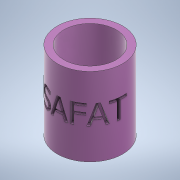
# Autodesk Inventor part: Repujado 2
Saved by Autodesk Inventor 2021 (Build 250183000, 183)
## iProperties
Created: 2021-01-13
Part Number: Repujado 2
Material: Genérico
Document SubType Name: Modeling
Designer: yosaf
Density: 1 g/cm^3
Appearance: Valor por defecto
Author: yosaf
Autodesk Inventor part; units mm, degrees
ref_plane "YZ Plane" through (0, 0, 0) normal (1, 0, 0) x (0, 1, 0)
ref_plane "XZ Plane" through (0, 0, 0) normal (0, 1, 0) x (-1, 0, 0)
sketch "Boceto1" plane through (0, 0, 0) normal (0, 1, 0) x (-1, 0, 0)
  circle A0 centre (0, 0) radius 25
  dimension "d0" = 50
  constraints: 1 centre point, 1 coincident
  measures "d0" diameter of A0
extrude "Extrusión1" add sketch "Boceto1" along normal blind 60
ref_plane "Plano de trabajo1" through (0, 0, 25) normal (0, 0, 1) x (1, 0, 0)
sketch "Boceto2" plane through (0, 0, 25) normal (0, 0, 1) x (1, 0, 0)
  line L0 (-43.1881, 39.0863) -> (43.2155, 39.0863) construction
  line L1 (43.2155, 39.0863) -> (43.2155, 23.3552) construction
  line L2 (43.2155, 23.3552) -> (-43.1881, 23.3552) construction
  line L3 (-43.1881, 23.3552) -> (-43.1881, 39.0863) construction
  line L4 (-31.1662, 38.7702) -> (-36.2351, 30.4072)
  line L5 (-36.2351, 30.4072) -> (-36.2351, 23.7702)
  line L6 (-36.2351, 23.7702) -> (-38.2286, 23.7702)
  line L7 (-38.2286, 23.7702) -> (-38.2286, 30.2005)
  line L8 (-38.2286, 30.2005) -> (-43.2975, 38.7702)
  line L9 (-43.2975, 38.7702) -> (-41.0852, 38.7702)
  line L10 (-41.0852, 38.7702) -> (-37.2197, 32.1697)
  line L11 (-37.2197, 32.1697) -> (-33.2813, 38.7702)
  line L12 (-33.2813, 38.7702) -> (-31.1662, 38.7702)
  spline S0 degree 2 poles (-19.1687, 37.0563) (-18.3178, 36.0595) (-17.3696, 33.1422) (-17.3696, 31.2702) knots 0 0 0 1 2 2 2
  spline S1 degree 2 poles (-17.3696, 31.2702) (-17.3696, 29.4469) (-18.2935, 26.4931) (-19.1687, 25.4963) knots 0 0 0 1 2 2 2
  spline S2 degree 2 poles (-19.1687, 25.4963) (-20.0925, 24.4509) (-22.5358, 23.4542) (-24.0066, 23.4542) knots 0 0 0 1 2 2 2
  spline S3 degree 2 poles (-24.0066, 23.4542) (-25.526, 23.4542) (-27.9572, 24.4874) (-28.8445, 25.4963) knots 0 0 0 1 2 2 2
  spline S4 degree 2 poles (-28.8445, 25.4963) (-29.7076, 26.4931) (-30.6314, 29.4226) (-30.6314, 31.2702) knots 0 0 0 1 2 2 2
  spline S5 degree 2 poles (-30.6314, 31.2702) (-30.6314, 33.1543) (-29.6954, 36.0231) (-28.8324, 37.0563) knots 0 0 0 1 2 2 2
  spline S6 degree 2 poles (-28.8324, 37.0563) (-27.9572, 38.053) (-25.5139, 39.0863) (-24.0066, 39.0863) knots 0 0 0 1 2 2 2
  spline S7 degree 2 poles (-24.0066, 39.0863) (-22.475, 39.0863) (-20.0196, 38.0166) (-19.1687, 37.0563) knots 0 0 0 1 2 2 2
  spline S8 degree 2 poles (-19.4482, 31.2702) (-19.4482, 32.7532) (-20.0925, 35.0506) (-20.676, 35.8043) knots 0 0 0 1 2 2 2
  spline S9 degree 2 poles (-20.676, 35.8043) (-21.2716, 36.5822) (-22.949, 37.3602) (-23.9944, 37.3602) knots 0 0 0 1 2 2 2
  spline S10 degree 2 poles (-23.9944, 37.3602) (-25.0763, 37.3602) (-26.7051, 36.6065) (-27.3251, 35.8043) knots 0 0 0 1 2 2 2
  spline S11 degree 2 poles (-27.3251, 35.8043) (-27.9207, 35.0385) (-28.5528, 32.7289) (-28.5528, 31.2702) knots 0 0 0 1 2 2 2
  spline S12 degree 2 poles (-28.5528, 31.2702) (-28.5528, 28.3164) (-26.073, 25.1803) (-23.9944, 25.1803) knots 0 0 0 1 2 2 2
  spline S13 degree 2 poles (-23.9944, 25.1803) (-21.9158, 25.1803) (-19.4482, 28.3164) (-19.4482, 31.2702) knots 0 0 0 1 2 2 2
  spline S14 degree 2 poles (-11.0001, 23.5028) (-12.629, 23.5028) (-14.9142, 24.1835) (-15.9231, 24.6697) knots 0 0 0 1 2 2 2
  line L13 (-15.9231, 24.6697) -> (-15.9231, 27.1738)
  line L14 (-15.9231, 27.1738) -> (-15.7772, 27.1738)
  spline S15 degree 2 poles (-15.7772, 27.1738) (-14.7926, 26.25) (-12.3008, 25.2289) (-11.146, 25.2289) knots 0 0 0 1 2 2 2
  spline S16 degree 2 poles (-11.146, 25.2289) (-9.4928, 25.2289) (-7.8032, 26.6025) (-7.8032, 27.7329) knots 0 0 0 1 2 2 2
  spline S17 degree 2 poles (-7.8032, 27.7329) (-7.8032, 28.6325) (-8.6905, 29.7508) (-9.6508, 30.0304) knots 0 0 0 1 2 2 2
  spline S18 degree 2 poles (-9.6508, 30.0304) (-10.3437, 30.2248) (-11.4985, 30.4923) (-12.3615, 30.7111) knots 0 0 0 1 2 2 2
  spline S19 degree 2 poles (-12.3615, 30.7111) (-13.1395, 30.9177) (-14.3672, 31.5376) (-14.8413, 32.036) knots 0 0 0 1 2 2 2
  spline S20 degree 2 poles (-14.8413, 32.036) (-15.3032, 32.5344) (-15.8137, 33.8715) (-15.8137, 34.7467) knots 0 0 0 1 2 2 2
  spline S21 degree 2 poles (-15.8137, 34.7467) (-15.8137, 36.5701) (-12.9693, 39.0376) (-10.7691, 39.0376) knots 0 0 0 1 2 2 2
  spline S22 degree 2 poles (-10.7691, 39.0376) (-9.505, 39.0376) (-7.2683, 38.5393) (-6.308, 38.0652) knots 0 0 0 1 2 2 2
  line L15 (-6.308, 38.0652) -> (-6.308, 35.6827)
  line L16 (-6.308, 35.6827) -> (-6.4539, 35.6827)
  spline S23 degree 2 poles (-6.4539, 35.6827) (-7.1711, 36.3391) (-9.4077, 37.3115) (-10.6354, 37.3115) knots 0 0 0 1 2 2 2
  spline S24 degree 2 poles (-10.6354, 37.3115) (-12.0212, 37.3115) (-13.7351, 36.0109) (-13.7351, 34.9534) knots 0 0 0 1 2 2 2
  spline S25 degree 2 poles (-13.7351, 34.9534) (-13.7351, 34.0052) (-12.7262, 32.8748) (-11.7781, 32.6195) knots 0 0 0 1 2 2 2
  spline S26 degree 2 poles (-11.7781, 32.6195) (-11.146, 32.4493) (-9.3105, 32.0117) (-8.7027, 31.8294) knots 0 0 0 1 2 2 2
  spline S27 degree 2 poles (-8.7027, 31.8294) (-7.1589, 31.3553) (-5.7246, 29.4469) (-5.7246, 28.049) knots 0 0 0 1 2 2 2
  spline S28 degree 2 poles (-5.7246, 28.049) (-5.7246, 27.1616) (-6.4418, 25.4598) (-7.086, 24.8642) knots 0 0 0 1 2 2 2
  spline S29 degree 2 poles (-7.086, 24.8642) (-7.8032, 24.2078) (-9.6265, 23.5028) (-11.0001, 23.5028) knots 0 0 0 1 2 2 2
  line L17 (-5.3113, 23.7702) -> (-0.2546, 38.7702)
  line L18 (-0.2546, 38.7702) -> (2.2009, 38.7702)
  line L19 (2.2009, 38.7702) -> (7.2576, 23.7702)
  line L20 (7.2576, 23.7702) -> (5.1547, 23.7702)
  line L21 (5.1547, 23.7702) -> (3.7933, 27.9639)
  line L22 (3.7933, 27.9639) -> (-1.932, 27.9639)
  line L23 (-1.932, 27.9639) -> (-3.2935, 23.7702)
  line L24 (-3.2935, 23.7702) -> (-5.3113, 23.7702)
  line L25 (3.2463, 29.6657) -> (0.9245, 36.7281)
  line L26 (0.9245, 36.7281) -> (-1.385, 29.6657)
  line L27 (-1.385, 29.6657) -> (3.2463, 29.6657)
  line L28 (17.6506, 36.9955) -> (10.6733, 36.9955)
  line L29 (10.6733, 36.9955) -> (10.6733, 32.7654)
  line L30 (10.6733, 32.7654) -> (17.3589, 32.7654)
  line L31 (17.3589, 32.7654) -> (17.3589, 30.9906)
  line L32 (17.3589, 30.9906) -> (10.6733, 30.9906)
  line L33 (10.6733, 30.9906) -> (10.6733, 23.7702)
  line L34 (10.6733, 23.7702) -> (8.6798, 23.7702)
  line L35 (8.6798, 23.7702) -> (8.6798, 38.7702)
  line L36 (8.6798, 38.7702) -> (17.6506, 38.7702)
  line L37 (17.6506, 38.7702) -> (17.6506, 36.9955)
  line L38 (17.8208, 23.7702) -> (22.8775, 38.7702)
  line L39 (22.8775, 38.7702) -> (25.333, 38.7702)
  line L40 (25.333, 38.7702) -> (30.3897, 23.7702)
  line L41 (30.3897, 23.7702) -> (28.2868, 23.7702)
  line L42 (28.2868, 23.7702) -> (26.9253, 27.9639)
  line L43 (26.9253, 27.9639) -> (21.2001, 27.9639)
  line L44 (21.2001, 27.9639) -> (19.8386, 23.7702)
  line L45 (19.8386, 23.7702) -> (17.8208, 23.7702)
  line L46 (26.3783, 29.6657) -> (24.0566, 36.7281)
  line L47 (24.0566, 36.7281) -> (21.7471, 29.6657)
  line L48 (21.7471, 29.6657) -> (26.3783, 29.6657)
  line L49 (35.3127, 23.7702) -> (35.3127, 36.9955)
  line L50 (35.3127, 36.9955) -> (30.2803, 36.9955)
  line L51 (30.2803, 36.9955) -> (30.2803, 38.7702)
  line L52 (30.2803, 38.7702) -> (42.3386, 38.7702)
  line L53 (42.3386, 38.7702) -> (42.3386, 36.9955)
  line L54 (42.3386, 36.9955) -> (37.3062, 36.9955)
  line L55 (37.3062, 36.9955) -> (37.3062, 23.7702)
  line L56 (37.3062, 23.7702) -> (35.3127, 23.7702)
  point P0 (0, 0)
  constraints: 2 other
emboss "Repujado1" sketch "Boceto2" operation cut depth 3 direction (0, 0, -1) wrap yes faces at (-24.6763, 40, -4.0103)
sketch "Boceto3" plane through (0, 60, 0) normal (0, 1, 0) x (1, 0, 0)
  circle A0 centre (0, 0) radius 20
  dimension "d6" = 40
  constraints: 1 centre point, 1 coincident
  measures "d6" diameter of A0
extrude "Extrusión2" cut sketch "Boceto3" against normal blind 57
